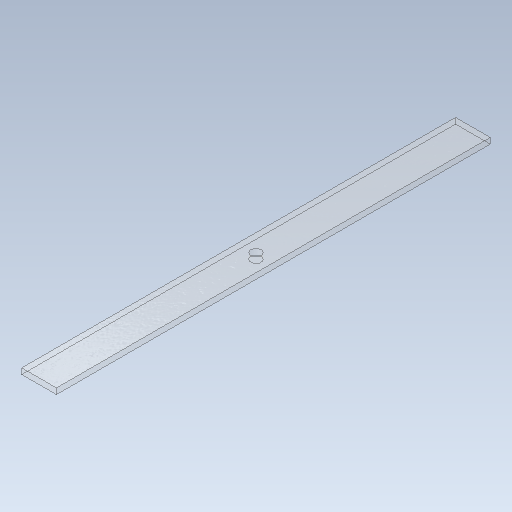
# Autodesk Inventor part: Base.pin.Seg
Saved by Autodesk Inventor 2020 (Build 240168000, 168)
## iProperties
Created: 2018-09-24
Part Number: Base.pin.Seg
Material: Acrílico, claro
Document SubType Name: Modeling
Designer: Cristiano
Density: 1.19 g/cm^3
Appearance: Transparente - Claro
Author: Cristiano
Autodesk Inventor part; units mm, degrees
ref_plane "YZ Plane" through (0, 0, 0) normal (1, 0, 0) x (0, 1, 0)
ref_plane "XZ Plane" through (0, 0, 0) normal (0, 1, 0) x (-1, 0, 0)
ref_plane "XY Plane" through (0, 0, 0) normal (0, 0, 1) x (1, 0, 0)
sketch "Boceto1" plane through (0, 0, 0) normal (0, 1, 0) x (-1, 0, 0)
  line L0 (0, 0) -> (30, 0)
  line L1 (30, 0) -> (30, -375)
  line L2 (30, -375) -> (0, -375)
  line L3 (0, -375) -> (0, 0)
  circle A0 centre (15, -187.5) radius 4.5
  dimension "d0" = 375
  dimension "d1" = 30
  dimension "d4" = 9
  dimension "d5" = 15
  dimension "d6" = 187.5
  constraints: 8 end point, 2 parallel, 1 centre point, 1 horizontal, 1 perpendicular
  measures "d0" distance of L0.end L1.end
  measures "d1" distance of L0.start L0.end
  measures "d4" diameter of A0
  measures "d5" distance from line of L1 A0.centre
  measures "d6" distance from line of L2 A0.centre
extrude "Extrusión2" add sketch "Boceto1" along normal blind 5
